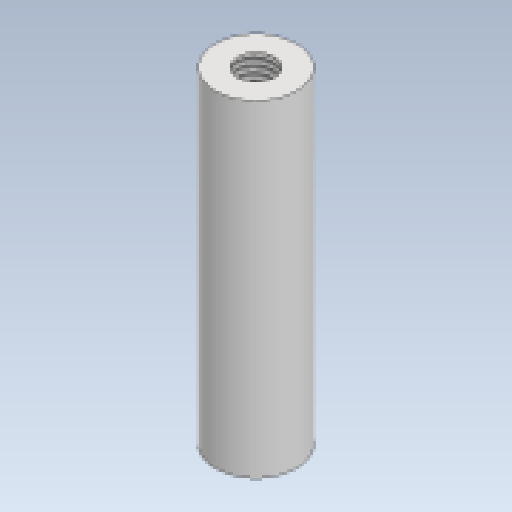
# Autodesk Inventor part: Support_bar
Saved by Autodesk Inventor 2025.2 (Build 292293000, 293)
## iProperties
Created: 2025-02-20
Part Number: Support_bar
Material: Generic
Document SubType Name: Modeling
Designer: Sergio Quintero
Density: 1 g/cm^3
Appearance: Default
Author: Sergio Quintero
Autodesk Inventor part; units mm, degrees
ref_plane "YZ Plane" through (0, 0, 0) normal (1, 0, 0) x (0, 1, 0)
ref_plane "XZ Plane" through (0, 0, 0) normal (0, 1, 0) x (-1, 0, 0)
ref_plane "XY Plane" through (0, 0, 0) normal (0, 0, 1) x (1, 0, 0)
sketch "Sketch1" plane through (0, 0, 0) normal (0, 1, 0) x (-1, 0, 0)
  circle A0 centre (0, 0) radius 7.5
  dimension "d0" = 15
  constraints: 1 centre point, 1 coincident
  measures "d0" diameter of A0
extrude "Extrusion1" add sketch "Sketch1" along normal blind 60
sketch "Sketch2" plane through (0, 60, 0) normal (0, 1, 0) x (1, 0, 0)
  circle A0 centre (0, 0) radius 7.5 projected
  constraints: 1 coincident
sketch "Sketch3" plane through (0, 0, 0) normal (0, -1, 0) x (1, 0, 0)
  point P0 (0, 0)
  point P1 (0, 0)
  constraints: 1 coincident
hole "Hole1" at (0, 60, 0) direction (0, -1, 0) diameter 6.647 depth 20 tip angle 118 thread size "M8x1.25" class "6H" standard "ISO Metric profile"
hole "Hole2" at (0, 0, 0) direction (0, 1, 0) diameter 6.647 depth 20 tip angle 118 thread size "M8x1.25" class "6H" standard "ISO Metric profile"
body "Solid1"
